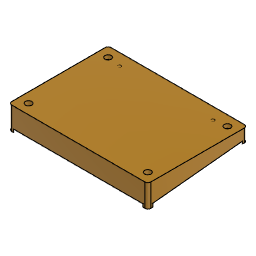
F24-Bottom (Autodesk Fusion 360 design; units mm, degrees)
Autodesk Fusion 360 part; units mm, degrees
note: some values were not read from the file. Chosen so that the rebuilt part matches the saved one: which face or edge a step refers to. Set by a fixed rule: which sketch regions a step uses.
sketch "Esquisse1" plane through (0, 0, 0) normal (0, 0, 1) x (1, 0, 0)
  line L0 (-70, 49.6722) -> (70, 49.6722)
  line L1 (70, 49.6722) -> (70, -50.3278)
  line L2 (70, -50.3278) -> (-70, -50.3278)
  line L3 (-70, -50.3278) -> (-70, 49.6722)
  line L4 (-65, 44.6722) -> (65, 44.6722)
  line L5 (65, 44.6722) -> (65, -45.3278)
  line L6 (65, -45.3278) -> (-65, -45.3278)
  line L7 (-65, -45.3278) -> (-65, 44.6722)
  line L8 (-50, 40) -> (50, 40)
  line L9 (50, 40) -> (50, -40)
  line L10 (50, -40) -> (-50, -40)
  line L11 (-50, -40) -> (-50, 40)
  line L12 (-50, 40) -> (50, -40) construction
  line L13 (50, 40) -> (-50, -40) construction
  circle A0 centre (-60, 39.6722) radius 5
  circle A1 centre (60, 39.6722) radius 5
  circle A2 centre (60, -40.3278) radius 5
  circle A3 centre (-60, -40.3278) radius 5
  circle A4 centre (-60, 39.6722) radius 1.6
  circle A5 centre (60, 39.6722) radius 1.6
  circle A6 centre (60, -40.3278) radius 1.6
  circle A7 centre (-60, -40.3278) radius 1.6
  line L14 (0, -50.3278) -> (0, 49.6722)
  circle A8 centre (-60, 39.6722) radius 3.2
  circle A9 centre (-60, -40.3278) radius 3.2
  circle A10 centre (60, 39.6722) radius 3.2
  circle A11 centre (60, -40.3278) radius 3.2
  line L15 (-65, -50.3278) -> (-70, -45.3278)
  line L16 (65, -50.3278) -> (70, -45.3278)
  line L17 (70, 44.6722) -> (65, 49.6722)
  line L18 (-70, 44.6722) -> (-65, 49.6722)
  line L19 (-60, -5) -> (60, -5)
  line L20 (60, -5) -> (60, -30.3)
  line L21 (60, -30.3) -> (-60, -30.3)
  line L22 (-60, -30.3) -> (-60, -5)
  line L23 (60, 5) -> (-60, 5)
  line L24 (-60, 5) -> (-60, 30.3)
  line L25 (-60, 30.3) -> (60, 30.3)
  line L26 (60, 30.3) -> (60, 5)
  point P0 (0, 49.6722)
  point P1 (-70, -0.3278)
  point P2 (70, -0.3278)
  point P3 (0, -50.3278)
  dimension "d5" = 140
  dimension "d6" = 100
  dimension "d11" = 5
  dimension "d12" = 5
  dimension "d13" = 5
  dimension "d14" = 5
  dimension "d15" = 80
  dimension "d16" = 100
  dimension "d17" = 10
  dimension "d18" = 10
  dimension "d19" = 10
  dimension "d20" = 10
  dimension "d21" = 3.2
  dimension "d22" = 3.2
  dimension "d23" = 3.2
  dimension "d24" = 3.2
  dimension "d84" = 6.4
  dimension "d85" = 6.4
  dimension "d86" = 6.4
  dimension "d87" = 6.4
  dimension "d96" = 5
  dimension "d97" = 5
  dimension "d98" = 5
  dimension "d99" = 5
  dimension "d100" = 5
  dimension "d101" = 5
  dimension "d102" = 5
  dimension "d107" = 25.3
  dimension "d108" = 25.3
  dimension "d109" = 5
  dimension "d110" = 5
  dimension "d111" = 5
  dimension "d112" = 5
  dimension "d113" = 5
  dimension "d114" = 5
  constraint horizontal L0
  constraint vertical L1
  constraint horizontal L2
  constraint vertical L3
  constraint midpoint L0 P0
  constraint midpoint L3 P1
  constraint midpoint L1 P2
  constraint midpoint L2 P3
  constraint horizontal L4
  constraint vertical L5
  constraint horizontal L6
  constraint vertical L7
  constraint horizontal L8
  constraint perpendicular L8 L9
  constraint parallel L8 L10
  constraint parallel L9 L11
  constraint coincident L12 origin
  constraint coincident L13 origin
  constraint tangent L4 A0
  constraint tangent L7 A0
  constraint tangent L4 A1
  constraint tangent L5 A1
  constraint tangent L5 A2
  constraint tangent L6 A2
  constraint tangent L7 A3
  constraint tangent L6 A3
  constraint concentric A0 A4
  constraint concentric A1 A5
  constraint concentric A2 A6
  constraint concentric A3 A7
  constraint coincident P3 L14.start
  constraint coincident P0 L14.end
  constraint concentric A0 A8
  constraint concentric A3 A9
  constraint concentric A1 A10
  constraint concentric A2 A11
  constraint coincident L2 L15.start
  constraint coincident L3 L15.end
  constraint coincident L2 L16.start
  constraint coincident L1 L16.end
  constraint coincident L1 L17.start
  constraint coincident L0 L17.end
  constraint perpendicular L16 L17
  constraint coincident L3 L18.start
  constraint coincident L0 L18.end
  constraint perpendicular L17 L18
  constraint horizontal L19
  constraint vertical L20
  constraint horizontal L21
  constraint vertical L22
  constraint horizontal L23
  constraint vertical L24
  constraint horizontal L25
  constraint vertical L26
  measures "d5" distance of L1 L3
  measures "d6" distance of L0 L2
  measures "d11" distance of L3 L7
  measures "d12" distance of L1 L5
  measures "d13" distance of L2 L6
  measures "d14" distance of L0 L4
  measures "d15" distance of L8 L10
  measures "d16" distance of L9 L11
  measures "d17" diameter of A0
  measures "d18" diameter of A3
  measures "d19" diameter of A2
  measures "d20" diameter of A1
  measures "d21" diameter of A4
  measures "d22" diameter of A5
  measures "d23" diameter of A6
  measures "d24" diameter of A7
  measures "d84" diameter of A8
  measures "d85" diameter of A10
  measures "d86" diameter of A11
  measures "d87" diameter of A9
  measures "d96" distance of L2.end L15.end
  measures "d97" distance of L2.end L15.start
  measures "d98" distance of L0.start L18.start
  measures "d99" distance of L0.start L18.end
  measures "d100" distance of L0.end L17.end
  measures "d101" distance of L0.end L17.start
  measures "d102" distance of L1.end L16.end
  measures "d107" distance of L19 L21
  measures "d108" distance of L23 L25
  measures "d109" distance of L7 L22
  measures "d110" distance of L5 L20
  measures "d111" distance of L7 L24
  measures "d112" distance of L5 L26
  measures "d113" distance of origin L19
  measures "d114" distance of origin L23
extrude "Extrusion1" add sketch "Esquisse1" along normal blind 3 contours L0 L3 L18 | L0 L2 L3 L4 L6 L7 L14 L15 L18 | L0 L1 L2 L4 L5 L6 L14 L16 L17 | L2 L3 L15 | L0 L1 L17 | L4 L6 L7 L8 L10 L11 A0 A3 L14 L19 L21 L22 L23 L24 L25 | L4 L5 L6 L8 L9 L10 A1 A2 L14 L19 L20 L21 L23 L25 L26 | L4 L7 A0 | A0 | L4 L5 A1 | A1 | L8 L11 L14 L25 | L8 L9 L14 L25 | L1 L2 L16 | L9 L14 L23 L25 | L11 L14 L23 L25 | L6 L7 A3 | A3 | A2 | L5 L6 A2 | L11 L23 L24 L25 | L9 L23 L25 L26 | L9 L14 L19 L23 | L11 L14 L19 L23 | L9 L10 L14 L21 | L10 L11 L14 L21 | L9 L14 L19 L21 | L11 L14 L19 L21 | L11 L19 L21 L22 | L9 L19 L20 L21 | A4 | A5 | A6 | A7 | A8 | A9 | A10 | A11
extrude "Extrusion2" add sketch "Esquisse1" against normal blind 3 contours L0 L3 L18 | L0 L2 L3 L4 L6 L7 L14 L15 L18 | L0 L1 L2 L4 L5 L6 L14 L16 L17 | L2 L3 L15 | L0 L1 L17 | L4 L6 L7 L8 L10 L11 A0 A3 L14 L19 L21 L22 L23 L24 L25 | L4 L5 L6 L8 L9 L10 A1 A2 L14 L19 L20 L21 L23 L25 L26 | L4 L7 A0 | A0 | L4 L5 A1 | A1 | L8 L11 L14 L25 | L8 L9 L14 L25 | L1 L2 L16 | L9 L14 L23 L25 | L11 L14 L23 L25 | L6 L7 A3 | A3 | A2 | L5 L6 A2 | L11 L23 L24 L25 | L9 L23 L25 L26 | L9 L14 L19 L23 | L11 L14 L19 L23 | L9 L10 L14 L21 | L10 L11 L14 L21 | L9 L14 L19 L21 | L11 L14 L19 L21 | L11 L19 L21 L22 | L9 L19 L20 L21 | A8 | A9 | A10 | A11
extrude "Extrusion3" add sketch "Esquisse1" against normal blind 17 contours L0 L3 L18 | L0 L2 L3 L4 L6 L7 L14 L15 L18 | L0 L1 L2 L4 L5 L6 L14 L16 L17 | L2 L3 L15 | L0 L1 L17 | L4 L7 A0 | A0 | L4 L5 A1 | A1 | L1 L2 L16 | L6 L7 A3 | A3 | A2 | L5 L6 A2 | A8 | A9 | A10 | A11
sketch "Esquisse3" plane through (-70, 0, 0) normal (-1, 0, 0) x (0, -1, 0)
  line L0 (50.3278, -17) -> (50.3278, 3)
  line L1 (50.3278, 3) -> (-49.6722, 3)
  line L2 (-49.6722, 3) -> (-49.6722, -17)
  line L3 (-49.6722, -17) -> (50.3278, -17)
sketch "Esquisse4" plane through (70, 0, 0) normal (1, 0, 0) x (0, 1, 0)
  line L0 (49.6722, -17) -> (49.6722, 3)
  line L1 (49.6722, 3) -> (-50.3278, 3)
  line L2 (-50.3278, 3) -> (-50.3278, -17)
  line L3 (-50.3278, -17) -> (49.6722, -17)
  line L4 (-50.3278, -17) -> (49.6722, -7)
  line L5 (-50.3278, -7.4058) -> (-50.3278, -17)
  dimension "d32" = 10
  dimension "d33" = 2.862
  constraint coincident L2.end L3.start
  constraint coincident L0 L4.end
  constraint coincident L2 L5.start
  constraint perpendicular L3 L5
  measures "d32" distance of L0.start L4.end
sketch "Esquisse6" plane through (0, 0, -17) normal (0, 0, -1) x (1, 0, 0)
  circle A0 centre (-60, -39.6722) radius 1.6
  circle A1 centre (60, -39.6722) radius 1.6
  line L0 (-60, 45.3278) -> (60, 45.3278)
  arc A2 (60, 45.3278) -> (65, 40.3278) centre (60, 40.3278) ccw
  line L1 (65, 40.3278) -> (65, -39.6722)
  arc A3 (65, -39.6722) -> (60, -44.6722) centre (60, -39.6722) ccw
  line L2 (60, -44.6722) -> (-60, -44.6722)
  arc A4 (-60, -44.6722) -> (-65, -39.6722) centre (-60, -39.6722) ccw
  line L3 (-65, -39.6722) -> (-65, 40.3278)
  arc A5 (-65, 40.3278) -> (-60, 45.3278) centre (-60, 40.3278) ccw
  circle A6 centre (60, 40.3278) radius 1.6
  circle A7 centre (-60, 40.3278) radius 1.6
  line L4 (70, 50.3278) -> (-70, 50.3278)
  line L5 (-70, 50.3278) -> (-70, -49.6722)
  line L6 (-70, -49.6722) -> (70, -49.6722)
  line L7 (70, -49.6722) -> (70, 50.3278)
  circle A8 centre (-60, 40.3278) radius 3.3
  circle A9 centre (-60, -39.6722) radius 3.3
  circle A10 centre (60, -39.6722) radius 3.3
  circle A11 centre (60, 40.3278) radius 3.3
  line L8 (-59.9911, 43.6278) -> (-62.8534, 41.9855)
  line L9 (-62.8534, 41.9855) -> (-62.8623, 38.6855)
  line L10 (-62.8623, 38.6855) -> (-60.0089, 37.0278)
  line L11 (-60.0089, 37.0278) -> (-57.1466, 38.6701)
  line L12 (-57.1466, 38.6701) -> (-57.1377, 41.9701)
  line L13 (-57.1377, 41.9701) -> (-59.9911, 43.6278)
  line L14 (59.9911, 43.6278) -> (57.1377, 41.9701)
  line L15 (57.1377, 41.9701) -> (57.1466, 38.6701)
  line L16 (57.1466, 38.6701) -> (60.0089, 37.0278)
  line L17 (60.0089, 37.0278) -> (62.8623, 38.6855)
  line L18 (62.8623, 38.6855) -> (62.8534, 41.9855)
  line L19 (62.8534, 41.9855) -> (59.9911, 43.6278)
  line L20 (59.9911, -36.3722) -> (57.1377, -38.0299)
  line L21 (57.1377, -38.0299) -> (57.1466, -41.3299)
  line L22 (57.1466, -41.3299) -> (60.0089, -42.9722)
  line L23 (60.0089, -42.9722) -> (62.8623, -41.3145)
  line L24 (62.8623, -41.3145) -> (62.8534, -38.0145)
  line L25 (62.8534, -38.0145) -> (59.9911, -36.3722)
  line L26 (-60, -36.3722) -> (-62.8579, -38.0222)
  line L27 (-62.8579, -38.0222) -> (-62.8579, -41.3222)
  line L28 (-62.8579, -41.3222) -> (-60, -42.9722)
  line L29 (-60, -42.9722) -> (-57.1421, -41.3222)
  line L30 (-57.1421, -41.3222) -> (-57.1421, -38.0222)
  line L31 (-57.1421, -38.0222) -> (-60, -36.3722)
  point P0 (-60, 40.3278)
  point P1 (60, 40.3278)
  point P2 (60, -39.6722)
  point P3 (-60, -39.6722)
  point P4 (-60, -39.6722)
  dimension "d38" = 6.6
  dimension "d39" = 6.6
  dimension "d40" = 6.6
  dimension "d41" = 6.6
  constraint concentric A5 A8
  constraint concentric A0 A9
  constraint concentric A1 A10
  constraint concentric A2 A11
  constraint coincident A8 L8.start
  constraint coincident P0 A5.centre
  constraint coincident A11 L14.start
  constraint coincident P1 A2.centre
  constraint coincident P2 A1.centre
  constraint coincident A10 L20.start
  constraint coincident P4 P3
  constraint coincident A9 L26.start
  measures "d38" diameter of A8
  measures "d39" diameter of A9
  measures "d40" diameter of A10
  measures "d41" diameter of A11
extrude "Extrusion6" cut sketch "Esquisse6" against normal blind 11.6 contours A0 | A1 | L26 L27 L28 L29 L30 L31 | L20 L21 L22 L23 L24 L25
extrude "Extrusion7" cut sketch "Esquisse6" against normal blind 3.6 contours A6 | A7 | L8 L9 L10 L11 L12 L13 | L14 L15 L16 L17 L18 L19
extrude "Extrusion8" cut sketch "Esquisse4" against normal blind 163 contours L0 L3 L4
sketch "Esquisse5" plane through (0, 0.7589, -8.4317) normal (0, 0.089638, -0.995974) x (-1, 0, 0)
  line L0 (70, -50.964) -> (70, 49.4402)
  line L1 (70, 49.4402) -> (-70, 49.4402)
  line L2 (-70, 49.4402) -> (-70, -50.964)
  line L3 (-70, -50.964) -> (70, -50.964)
  ellipse E0 centre (60, -40.9236) end of major axis (60, -42.9317) minor radius 2
  ellipse E1 centre (-60, -40.9236) end of major axis (-60, -42.9317) minor radius 2
  ellipse E2 centre (60, 39.3998) end of major axis (60, 37.3917) minor radius 2
  ellipse E3 centre (-60, 39.3998) end of major axis (-60, 37.3917) minor radius 2
  line L4 (-60, 44.42) -> (60, 44.42)
  ellipse E4 centre (60, 39.3998) end of major axis (60, 34.3795) minor radius 5 (60, 44.42) -> (65, 39.3998) ccw
  line L5 (65, 39.3998) -> (65, -40.9236)
  ellipse E5 centre (60, -40.9236) end of major axis (60, -45.9438) minor radius 5 (65, -40.9236) -> (60, -45.9438) ccw
  line L6 (60, -45.9438) -> (-60, -45.9438)
  ellipse E6 centre (-60, -40.9236) end of major axis (-60, -45.9438) minor radius 5 (-60, -45.9438) -> (-65, -40.9236) ccw
  line L7 (-65, -40.9236) -> (-65, 39.3998)
  ellipse E7 centre (-60, 39.3998) end of major axis (-60, 34.3795) minor radius 5 (-65, 39.3998) -> (-60, 44.42) ccw
sketch "Esquisse7" plane through (0, 1.1849, -11.8487) normal (0, 0.099504, -0.995037) x (-1, 0, 0)
  line L0 (70, -51.7696) -> (70, 48.7292)
  line L1 (70, 48.7292) -> (-70, 48.7292)
  line L2 (-70, 48.7292) -> (-70, -51.7696)
  line L3 (-70, -51.7696) -> (70, -51.7696)
  line L4 (-60, 43.7042) -> (60, 43.7042)
  ellipse E0 centre (60, 38.6793) end of major axis (60, 33.6543) minor radius 5 (60, 43.7042) -> (65, 38.6793) ccw
  line L5 (65, 38.6793) -> (65, -41.7197)
  ellipse E1 centre (60, -41.7197) end of major axis (60, -46.7447) minor radius 5 (65, -41.7197) -> (60, -46.7447) ccw
  line L6 (60, -46.7447) -> (-60, -46.7447)
  ellipse E2 centre (-60, -41.7197) end of major axis (-60, -46.7447) minor radius 5 (-60, -46.7447) -> (-65, -41.7197) ccw
  line L7 (-65, -41.7197) -> (-65, 38.6793)
  ellipse E3 centre (-60, 38.6793) end of major axis (-60, 33.6543) minor radius 5 (-65, 38.6793) -> (-60, 43.7042) ccw
  line L8 (-57.1377, 37.0288) -> (-59.9911, 35.3628)
  line L9 (-59.9911, 35.3628) -> (-62.8534, 37.0133)
  line L10 (-62.8534, 37.0133) -> (-62.8623, 40.3298)
  line L11 (-62.8623, 40.3298) -> (-60.0089, 41.9957)
  line L12 (-60.0089, 41.9957) -> (-57.1466, 40.3453)
  line L13 (-57.1466, 40.3453) -> (-57.1377, 37.0288)
  line L14 (-57.1377, -43.3702) -> (-59.9911, -45.0362)
  line L15 (-59.9911, -45.0362) -> (-62.8534, -43.3857)
  line L16 (-62.8534, -43.3857) -> (-62.8623, -40.0692)
  line L17 (-62.8623, -40.0692) -> (-60.0089, -38.4033)
  line L18 (-60.0089, -38.4033) -> (-57.1466, -40.0538)
  line L19 (-57.1466, -40.0538) -> (-57.1377, -43.3702)
  line L20 (62.8534, -43.3857) -> (59.9911, -45.0362)
  line L21 (59.9911, -45.0362) -> (57.1377, -43.3702)
  line L22 (57.1377, -43.3702) -> (57.1466, -40.0538)
  line L23 (57.1466, -40.0538) -> (60.0089, -38.4033)
  line L24 (60.0089, -38.4033) -> (62.8623, -40.0692)
  line L25 (62.8623, -40.0692) -> (62.8534, -43.3857)
  line L26 (49.9999, -40.9996) -> (-50.0001, -40.9996)
  line L27 (-50.0001, -40.9996) -> (-50.0001, 41.0004)
  line L28 (-50.0001, 41.0004) -> (49.9999, 41.0004)
  line L29 (49.9999, 41.0004) -> (49.9999, -40.9996)
  circle A0 centre (46.9999, -37.9996) radius 4
  circle A1 centre (-47.0001, -37.9996) radius 4
  circle A2 centre (-47.0001, 38.0004) radius 4
  circle A3 centre (46.9999, 38.0004) radius 4
  circle A4 centre (46.9999, -37.9996) radius 3.3
  circle A5 centre (-47.0001, -37.9996) radius 3.3
  circle A6 centre (-47.0001, 38.0004) radius 3.3
  circle A7 centre (46.9999, 38.0004) radius 3.3
  line L30 (-47.0001, 34.7004) -> (-44.1422, 36.3504)
  line L31 (-44.1422, 36.3504) -> (-44.1422, 39.6504)
  line L32 (-44.1422, 39.6504) -> (-47.0001, 41.3004)
  line L33 (-47.0001, 41.3004) -> (-49.858, 39.6504)
  line L34 (-49.858, 39.6504) -> (-49.858, 36.3504)
  line L35 (-49.858, 36.3504) -> (-47.0001, 34.7004)
  line L36 (46.9999, 34.7004) -> (49.8578, 36.3504)
  line L37 (49.8578, 36.3504) -> (49.8578, 39.6504)
  line L38 (49.8578, 39.6504) -> (46.9999, 41.3004)
  line L39 (46.9999, 41.3004) -> (44.142, 39.6504)
  line L40 (44.142, 39.6504) -> (44.142, 36.3504)
  line L41 (44.142, 36.3504) -> (46.9999, 34.7004)
  circle A8 centre (-47.0001, 38.0004) radius 1.6
  circle A9 centre (46.9999, 38.0004) radius 1.6
  circle A10 centre (46.9999, -37.9996) radius 1.6
  circle A11 centre (-47.0001, -37.9996) radius 1.6
  line L42 (-0.0001, 41.0004) -> (-0.0001, -40.9996)
  line L43 (-50.0001, 0.0004) -> (49.9999, 0.0004)
  line L44 (46.9999, -34.6996) -> (44.142, -36.3496)
  line L45 (44.142, -36.3496) -> (44.142, -39.6496)
  line L46 (44.142, -39.6496) -> (46.9999, -41.2996)
  line L47 (46.9999, -41.2996) -> (49.8578, -39.6496)
  line L48 (49.8578, -39.6496) -> (49.8578, -36.3496)
  line L49 (49.8578, -36.3496) -> (46.9999, -34.6996)
  line L50 (-47.0001, -34.6996) -> (-49.858, -36.3496)
  line L51 (-49.858, -36.3496) -> (-49.858, -39.6496)
  line L52 (-49.858, -39.6496) -> (-47.0001, -41.2996)
  line L53 (-47.0001, -41.2996) -> (-44.1422, -39.6496)
  line L54 (-44.1422, -39.6496) -> (-44.1422, -36.3496)
  line L55 (-44.1422, -36.3496) -> (-47.0001, -34.6996)
  line L56 (60, 41.9957) -> (62.8579, 40.3375)
  line L57 (62.8579, 40.3375) -> (62.8579, 37.0211)
  line L58 (62.8579, 37.0211) -> (60, 35.3628)
  line L59 (60, 35.3628) -> (57.1421, 37.0211)
  line L60 (57.1421, 37.0211) -> (57.1421, 40.3375)
  line L61 (57.1421, 40.3375) -> (60, 41.9957)
  point P0 (49.9999, 0.0004)
  point P1 (-50.0001, 0.0004)
  point P2 (-0.0001, -40.9996)
  point P3 (-0.0001, 41.0004)
  point P4 (-47.0001, 38.0004)
  point P5 (46.9999, 38.0004)
  point P6 (46.9999, -37.9996)
  point P7 (-47.0001, -37.9996)
  point P8 (46.9999, -37.9996)
  point P9 (-47.0001, -37.9996)
  dimension "d48" = 100
  dimension "d49" = 82
  dimension "d50" = 3
  dimension "d51" = 3
  dimension "d52" = 3
  dimension "d53" = 3
  dimension "d54" = 3
  dimension "d55" = 3
  dimension "d56" = 3
  dimension "d57" = 3
  dimension "d58" = 8
  dimension "d59" = 8
  dimension "d60" = 8
  dimension "d61" = 8
  dimension "d66" = 6.6
  dimension "d67" = 6.6
  dimension "d68" = 6.6
  dimension "d69" = 6.6
  dimension "d70" = 3.2
  dimension "d71" = 3.2
  dimension "d72" = 3.2
  dimension "d73" = 3.2
  dimension "d130" = 20.0001
  dimension "d131" = 7.7287
  constraint horizontal L26
  constraint vertical L27
  constraint horizontal L28
  constraint vertical L29
  constraint midpoint L29 P0
  constraint midpoint L27 P1
  constraint midpoint L26 P2
  constraint midpoint L28 P3
  constraint concentric A0 A4
  constraint concentric A1 A5
  constraint concentric A2 A6
  constraint concentric A3 A7
  constraint coincident A6 L30.start
  constraint coincident P4 A2.centre
  constraint coincident P5 A3.centre
  constraint coincident A7 L36.start
  constraint coincident P8 P6
  constraint coincident P9 P7
  constraint concentric A6 A8
  constraint concentric A4 A10
  constraint concentric A1 A11
  constraint coincident P3 L42.start
  constraint coincident P2 L42.end
  constraint coincident P1 L43.start
  constraint coincident P0 L43.end
  constraint coincident A4 L44.start
  constraint coincident A5 L50.start
  measures "d48" distance of L27 L29
  measures "d49" distance of L26 L28
  measures "d50" distance of L26 P8
  measures "d51" distance of L29 P8
  measures "d52" distance of L27 P9
  measures "d53" distance of L26 P9
  measures "d54" distance of L29 P5
  measures "d55" distance of L28 P5
  measures "d56" distance of L28 P4
  measures "d57" distance of L27 P4
  measures "d58" diameter of A0
  measures "d59" diameter of A1
  measures "d60" diameter of A2
  measures "d61" diameter of A3
  measures "d66" diameter of A7
  measures "d67" diameter of A4
  measures "d68" diameter of A5
  measures "d69" diameter of A6
  measures "d70" diameter of A11
  measures "d71" diameter of A8
  measures "d72" diameter of A9
  measures "d73" diameter of A10
  measures "d130" distance of L0 L29
  measures "d131" distance of L1 L28
extrude "Extrusion9" add sketch "Esquisse7" against normal blind 10 contours L28 L29 A3 A7 | L29 A3 A7 | L27 L28 A2 A6 | L28 A2 A6 | L28 A3 A7 | L27 A2 A6 | L29 A7 L37 | L29 A7 | L28 A6 L32 | L28 A6 L32 | L27 L28 A2 A6 | L28 A7 L39 | L28 A7 L39 | L28 L29 A3 A7 | L27 A6 | L27 A6 L34 | A7 L36 | L28 L36 L37 L38 L39 L40 L41 | L28 L30 L31 L32 L33 L34 L35 | L28 L32 L33 | A6 L31 | L28 A6 L33 | L28 A6 L33 | L28 L38 L39 | L28 A7 L38 | A7 L40 | L28 A7 L38 | A6 L35 | A7 L41 | A6 L30 | A8 | A9
extrude "Extrusion10" add sketch "Esquisse7" against normal blind 15 contours L26 A0 A4 | L26 L29 A0 A4 | L29 A0 A4 | L26 A4 L47 | L26 A4 L47 | L26 L29 A0 A4 | L29 A4 L48 | L29 A4 | L26 L46 L47 | L26 L44 L45 L46 L47 L48 L49 | L26 A4 L46 | L26 A4 L46 | A4 L49 | A4 L45 | L26 A1 A5 | L26 L27 A1 A5 | A4 L44 | L26 A5 L53 | L26 A5 L53 | L26 L27 A1 A5 | L26 L52 L53 | L26 L50 L51 L52 L53 L54 L55 | L26 A5 L52 | A5 L54 | L26 A5 L52 | L27 A1 A5 | A5 L55 | L27 A5 L51 | L27 A5 | A5 L50 | A10 | A11
extrude "Extrusion11" cut sketch "Esquisse7" against normal blind 2.3 contours L28 L36 L37 L38 L39 L40 L41 | L28 L30 L31 L32 L33 L34 L35 | L28 L32 L33 | L28 L38 L39 | A8 | A9
extrude "Extrusion12" cut sketch "Esquisse7" against normal blind 2.3 contours L26 L50 L51 L52 L53 L54 L55 | L27 A1 A5 | L28 L30 L31 L32 L33 L34 L35 | L28 L32 L33 | A8 | A11
extrude "Extrusion13" cut sketch "Esquisse7" against normal blind 2.3 contours L26 L44 L45 L46 L47 L48 L49 | A10
extrude "Extrusion14" cut sketch "Esquisse7" against normal blind 10.5 contours A8 | A9
extrude "Extrusion15" cut sketch "Esquisse7" against normal blind 16 contours A10 | A11
extrude "Extrusion16" cut sketch "Esquisse1" along normal blind 5 and the other way blind 1 contours A4 | A5 | A8 | A10
extrude "Extrusion17" cut sketch "Esquisse1" along normal blind -9 and the other way blind -5 contours A6 | A7 | A9 | A11
extrude "Extrusion18" add sketch "Esquisse1" against normal blind 20 contours L2 L3 L15 | L1 L2 L16
extrude "Extrusion19" add sketch "Esquisse1" against normal blind 10 contours L0 L3 L18 | L0 L1 L17
extrude "Extrusion20" cut sketch "Esquisse1" against normal blind 3 contours L9 L14 L23 L25 | L11 L14 L23 L25 | L11 L23 L24 L25 | L9 L23 L25 L26 | L9 L14 L19 L21 | L11 L14 L19 L21 | L11 L19 L21 L22 | L9 L19 L20 L21
fillet "Congé1" radius 3 1 edges at (-70, -50.3278, -8.5)
fillet "Congé2" radius 3 1 edges at (-70, 49.6722, -3.5)
fillet "Congé3" radius 3 2 edges at (70, 49.6722, -3.5) (70, -50.3278, -8.5)
extrude "Extrusion5" cut sketch "Esquisse1" along normal blind 10 contours A4 | A5 | A6 | A7
extrude "Extrusion21" add 1 faces at (50.4881, -35.4633, -13.2021) along direction (0, 0.099504, -0.995037) blind 2.3
extrude "Extrusion22" cut sketch "Esquisse7" against normal blind 2.3 contours L26 L46 L47 | L26 L52 L53
chamfer "Chanfrein1" distance 2.5 distance2 1.6 4 edges at (58.5083, -40.9064, -9) (-61.4917, -40.9064, -9) (-61.4917, 39.0936, -1) (58.5083, 39.0936, -1) measured on face at (60.934, -39.0287, -11.9333) measured on face at (-59.066, -39.0287, -11.9333) measured on face at (-59.1319, 41.0162, -3.9333) measured on face at (60.8681, 41.0162, -3.9333)
move_body "Déplacer1" bodies 1 to x (1, 0, 0) y (0, 1, 0) z (0, 0, 1) at (0, 0, 6)
move_body "Déplacer2" bodies 1 to x (1, 0, 0) y (0, 1, 0) z (0, 0, 1) at (0, 0, 0)
equation "d42 = -12.5 mm + 0.9 mm"
